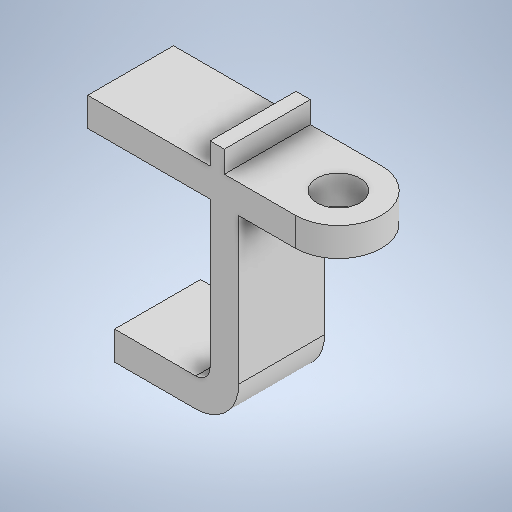
# Autodesk Inventor part: j1 endstop block v2
Saved by Autodesk Inventor 2025 (Build 290162000, 162)
## iProperties
Created: 2025-07-11
Part Number: j1 endstop block v2
Material: 一般
Document SubType Name: Modeling
Designer: gavin
Density: 1 g/cm^3
Appearance: 預設
Author: gavin
## iProperties of the stored document j1 endstop block v2_3D 列印.ipt
Created: 2025-07-11
Part Number: j1 endstop block v2_3D 列印
Material: 一般
Document SubType Name: Modeling
Designer: gavin
Density: 1 g/cm^3
Appearance: 預設
Author: gavin
Autodesk Inventor part; units mm, degrees
ref_plane "YZ Plane" through (0, 0, 0) normal (1, 0, 0) x (0, 1, 0)
ref_plane "XZ Plane" through (0, 0, 0) normal (0, 1, 0) x (-1, 0, 0)
sketch "草圖1" plane through (0, 0, 0) normal (0, 0, 1) x (1, 0, 0)
  line L0 (0, -6) -> (0.94, -6) construction
  line L1 (0, 0) -> (0, -6) construction
  line L2 (0.94, 0) -> (0, 0) projected
  line L3 (0.94, 0) -> (0.94, -6) construction
  line L4 (4.44, 0) -> (4.44, -6)
  line L5 (7.44, 0) -> (7.44, -6)
  line L6 (7.44, -6) -> (4.44, -6) projected
  line L7 (-0.03, -6) -> (-0.03, -4.4819)
  line L8 (-0.03, -4.4819) -> (0.97, -4.4819)
  line L9 (0.97, -4.4819) -> (0.97, -6)
  line L10 (0.97, -6) -> (8.94, -6)
  line L11 (8.94, -6) -> (8.94, -8)
  line L12 (8.94, -8) -> (-6.6252, -8)
  line L13 (-6.6252, -8) -> (-8.58, -8)
  line L14 (-8.58, -8) -> (-8.58, -6)
  line L15 (-8.58, -6) -> (-0.03, -6)
  line L16 (-9.58, -22.94) -> (-9.58, -18)
  point P0 (0.47, -6)
  point P1 (-8.58, -7)
  dimension "d0" = 1
  dimension "d1" = 0.03
  dimension "d2" = 0.94
  dimension "d3" = 1.5
  dimension "d5" = 2
  dimension "d18" = 1
  constraints: 24 end point, 7 perpendicular, 4 vertical, 3 point on line, 2 midpoint, 6 other
  measures "d0" distance of L7.end L8.end
  measures "d1" distance between parallel lines of L9 L3
  measures "d2" distance of L0.start L0.end
  measures "d3" distance between parallel lines of L5 L11
  measures "d5" distance of L10.end L11.end
  measures "d18" distance from line of L16 point (-8.58, -7)
extrude "擠出1" add sketch "草圖1" along normal up to surface (6 mm away)
ref_plane "工作平面1" through (-1.62, -18, -3) normal (1, 0, 0) x (0, 1, 0)
sketch "草圖3" plane through (0.97, -6, 0) normal (0, 1, 0) x (1, 0, 0)
  circle A0 centre (4.97, -3) radius 1.5 projected
  point P0 (-0.97, 0)
extrude "擠出3" cut sketch "草圖3" against normal up to surface (2 mm away)
fillet "圓角1" radius 3 2 edges at (8.94, -7, 6) (8.94, -7, 0)
sketch "草圖9" plane through (-8.58, -6, 6) normal (0, 0, 1) x (1, 0, 0)
  line L0 (14.52, 0) -> (14.52, -2) projected
  line L1 (9.55, 0) -> (14.52, 0) projected
  line L2 (9.55, 1.5181) -> (9.55, 0) projected
  line L3 (8.55, 1.5181) -> (9.55, 1.5181) projected
  line L4 (8.55, 0) -> (8.55, 1.5181) projected
  line L5 (0, 0) -> (8.55, 0) projected
  line L6 (0, -2) -> (0, 0) projected
  line L7 (14.52, -2) -> (0, -2) projected
  line L8 (-1, -12) -> (6.96, -12) projected
  line L9 (6.96, -12) -> (6.96, -8) projected
  line L10 (6.96, -8) -> (-2.84, -8) projected
  line L11 (-2.84, -20.94) -> (-2.84, -8) projected
  line L12 (-2.84, -20.94) -> (6.96, -20.94) projected
  line L13 (6.96, -20.94) -> (6.96, -16.94) projected
  line L14 (6.96, -16.94) -> (-1, -16.94) projected
  line L15 (-1, -16.94) -> (-1, -12) projected
  line L16 (1.884, -15.2) -> (1.884, -13.2)
  line L17 (1.884, -13.2) -> (8.55, -13.2)
  line L18 (8.55, -13.2) -> (8.55, -2)
  line L19 (1.884, -15.2) -> (10.55, -15.2)
  line L20 (10.55, -15.2) -> (10.55, -2)
  point P0 (8.58, 6)
  dimension "d28" = 2
  dimension "d29" = 2
  dimension "d30" = 1.2
  constraints: 10 end point, 3 perpendicular, 3 point on line, 1 horizontal, 1 vertical
  measures "d28" distance between parallel lines of L19 L17
  measures "d29" distance between parallel lines of L20 L18
  measures "d30" distance between parallel lines of L8 L17
extrude "擠出8" add sketch "草圖9" against normal up to surface (6 mm away) contours L20 L19 L16 L17 L18 L7
fillet "圓角2" radius 1 1 edges at (-0.03, -19.2, 3)
fillet "圓角3" radius 3 1 edges at (1.97, -21.2, 3)
equation "\"d1\" = -0.5 * d2 + 0.5 * d0"
